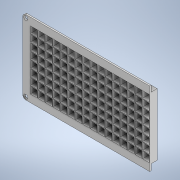
# Autodesk Inventor part: Grid
Saved by Autodesk Inventor 2020 (Build 240168000, 168)
## iProperties
Created: 2021-04-13
Part Number: Grid
Material: Generic
Document SubType Name: Modeling
Designer: user
Density: 1 g/cm^3
Appearance: Default
Author: user
Autodesk Inventor part; units mm, degrees
(part 1 of 2)
ref_plane "YZ Plane" through (0, 0, 0) normal (1, 0, 0) x (0, 1, 0)
ref_plane "XZ Plane" through (0, 0, 0) normal (0, 1, 0) x (-1, 0, 0)
ref_plane "XY Plane" through (0, 0, 0) normal (0, 0, 1) x (1, 0, 0)
sketch "Sketch4" plane through (0, 0, 0) normal (0, 0, 1) x (1, 0, 0)
  line L0 (0, 0) -> (5, 0)
  line L1 (5, 0) -> (5, 5)
  line L2 (5, 5) -> (0, 5)
  line L3 (0, 5) -> (0, 0)
  line L4 (-2, 7) -> (7, 7)
  line L5 (7, 7) -> (7, -2)
  line L6 (7, -2) -> (-2, -2)
  line L7 (-2, -2) -> (-2, 7)
  line L8 (10, 0) -> (15, 0)
  line L9 (15, 0) -> (15, 5)
  line L10 (15, 5) -> (10, 5)
  line L11 (10, 5) -> (10, 0)
  line L12 (20, 0) -> (25, 0)
  line L13 (25, 0) -> (25, 5)
  line L14 (25, 5) -> (20, 5)
  line L15 (20, 5) -> (20, 0)
  line L16 (30, 0) -> (35, 0)
  line L17 (35, 0) -> (35, 5)
  line L18 (35, 5) -> (30, 5)
  line L19 (30, 5) -> (30, 0)
  line L20 (40, 0) -> (45, 0)
  line L21 (45, 0) -> (45, 5)
  line L22 (45, 5) -> (40, 5)
  line L23 (40, 5) -> (40, 0)
  line L24 (50, 0) -> (55, 0)
  line L25 (55, 0) -> (55, 5)
  line L26 (55, 5) -> (50, 5)
  line L27 (50, 5) -> (50, 0)
  line L28 (60, 0) -> (65, 0)
  line L29 (65, 0) -> (65, 5)
  line L30 (65, 5) -> (60, 5)
  line L31 (60, 5) -> (60, 0)
  line L32 (70, 0) -> (75, 0)
  line L33 (75, 0) -> (75, 5)
  line L34 (75, 5) -> (70, 5)
  line L35 (70, 5) -> (70, 0)
  line L36 (80, 0) -> (85, 0)
  line L37 (85, 0) -> (85, 5)
  line L38 (85, 5) -> (80, 5)
  line L39 (80, 5) -> (80, 0)
  line L40 (90, 0) -> (95, 0)
  line L41 (95, 0) -> (95, 5)
  line L42 (95, 5) -> (90, 5)
  line L43 (90, 5) -> (90, 0)
  line L44 (100, 0) -> (105, 0)
  line L45 (105, 0) -> (105, 5)
  line L46 (105, 5) -> (100, 5)
  line L47 (100, 5) -> (100, 0)
  line L48 (110, 0) -> (115, 0)
  line L49 (115, 0) -> (115, 5)
  line L50 (115, 5) -> (110, 5)
  line L51 (110, 5) -> (110, 0)
  line L52 (120, 0) -> (125, 0)
  line L53 (125, 0) -> (125, 5)
  line L54 (125, 5) -> (120, 5)
  line L55 (120, 5) -> (120, 0)
  line L56 (130, 0) -> (135, 0)
  line L57 (135, 0) -> (135, 5)
  line L58 (135, 5) -> (130, 5)
  line L59 (130, 5) -> (130, 0)
  line L60 (140, 0) -> (145, 0)
  line L61 (145, 0) -> (145, 5)
  line L62 (145, 5) -> (140, 5)
  line L63 (140, 5) -> (140, 0)
  line L64 (150, 0) -> (155, 0)
  line L65 (155, 0) -> (155, 5)
  line L66 (155, 5) -> (150, 5)
  line L67 (150, 5) -> (150, 0)
  line L68 (160, 0) -> (165, 0)
  line L69 (165, 0) -> (165, 5)
  line L70 (165, 5) -> (160, 5)
  line L71 (160, 5) -> (160, 0)
  line L72 (170, 0) -> (175, 0)
  line L73 (175, 0) -> (175, 5)
  line L74 (175, 5) -> (170, 5)
  line L75 (170, 5) -> (170, 0)
  line L76 (180, 0) -> (185, 0)
  line L77 (185, 0) -> (185, 5)
  line L78 (185, 5) -> (180, 5)
  line L79 (180, 5) -> (180, 0)
  line L80 (190, 0) -> (195, 0)
  line L81 (195, 0) -> (195, 5)
  line L82 (195, 5) -> (190, 5)
  line L83 (190, 5) -> (190, 0)
  line L84 (200, 0) -> (205, 0)
  line L85 (205, 0) -> (205, 5)
  line L86 (205, 5) -> (200, 5)
  line L87 (200, 5) -> (200, 0)
  line L88 (210, 0) -> (215, 0)
  line L89 (215, 0) -> (215, 5)
  line L90 (215, 5) -> (210, 5)
  line L91 (210, 5) -> (210, 0)
  line L92 (220, 0) -> (225, 0)
  line L93 (225, 0) -> (225, 5)
  line L94 (225, 5) -> (220, 5)
  line L95 (220, 5) -> (220, 0)
  line L96 (230, 0) -> (235, 0)
  line L97 (235, 0) -> (235, 5)
  line L98 (235, 5) -> (230, 5)
  line L99 (230, 5) -> (230, 0)
  line L100 (240, 0) -> (245, 0)
  line L101 (245, 0) -> (245, 5)
  line L102 (245, 5) -> (240, 5)
  line L103 (240, 5) -> (240, 0)
  line L104 (250, 0) -> (255, 0)
  line L105 (255, 0) -> (255, 5)
  line L106 (255, 5) -> (250, 5)
  line L107 (250, 5) -> (250, 0)
  line L108 (260, 0) -> (265, 0)
  line L109 (265, 0) -> (265, 5)
  line L110 (265, 5) -> (260, 5)
  line L111 (260, 5) -> (260, 0)
  line L112 (270, 0) -> (275, 0)
  line L113 (275, 0) -> (275, 5)
  line L114 (275, 5) -> (270, 5)
  line L115 (270, 5) -> (270, 0)
  line L116 (280, 0) -> (285, 0)
  line L117 (285, 0) -> (285, 5)
  line L118 (285, 5) -> (280, 5)
  line L119 (280, 5) -> (280, 0)
  line L120 (290, 0) -> (295, 0)
  line L121 (295, 0) -> (295, 5)
  line L122 (295, 5) -> (290, 5)
  line L123 (290, 5) -> (290, 0)
  line L124 (300, 0) -> (305, 0)
  line L125 (305, 0) -> (305, 5)
  line L126 (305, 5) -> (300, 5)
  line L127 (300, 5) -> (300, 0)
  line L128 (310, 0) -> (315, 0)
  line L129 (315, 0) -> (315, 5)
  line L130 (315, 5) -> (310, 5)
  line L131 (310, 5) -> (310, 0)
  line L132 (0, -10) -> (5, -10)
  line L133 (5, -10) -> (5, -5)
  line L134 (5, -5) -> (0, -5)
  line L135 (0, -5) -> (0, -10)
  line L136 (10, -10) -> (15, -10)
  line L137 (15, -10) -> (15, -5)
  line L138 (15, -5) -> (10, -5)
  line L139 (10, -5) -> (10, -10)
  line L140 (20, -10) -> (25, -10)
  line L141 (25, -10) -> (25, -5)
  line L142 (25, -5) -> (20, -5)
  line L143 (20, -5) -> (20, -10)
  line L144 (30, -10) -> (35, -10)
  line L145 (35, -10) -> (35, -5)
  line L146 (35, -5) -> (30, -5)
  line L147 (30, -5) -> (30, -10)
  line L148 (40, -10) -> (45, -10)
  line L149 (45, -10) -> (45, -5)
  line L150 (45, -5) -> (40, -5)
  line L151 (40, -5) -> (40, -10)
  line L152 (50, -10) -> (55, -10)
  line L153 (55, -10) -> (55, -5)
  line L154 (55, -5) -> (50, -5)
  line L155 (50, -5) -> (50, -10)
  line L156 (60, -10) -> (65, -10)
  line L157 (65, -10) -> (65, -5)
  line L158 (65, -5) -> (60, -5)
  line L159 (60, -5) -> (60, -10)
  line L160 (70, -10) -> (75, -10)
  line L161 (75, -10) -> (75, -5)
  line L162 (75, -5) -> (70, -5)
  line L163 (70, -5) -> (70, -10)
  line L164 (80, -10) -> (85, -10)
  line L165 (85, -10) -> (85, -5)
  line L166 (85, -5) -> (80, -5)
  line L167 (80, -5) -> (80, -10)
  line L168 (90, -10) -> (95, -10)
  line L169 (95, -10) -> (95, -5)
  line L170 (95, -5) -> (90, -5)
  line L171 (90, -5) -> (90, -10)
  line L172 (100, -10) -> (105, -10)
  line L173 (105, -10) -> (105, -5)
  line L174 (105, -5) -> (100, -5)
  line L175 (100, -5) -> (100, -10)
  line L176 (110, -10) -> (115, -10)
  line L177 (115, -10) -> (115, -5)
  line L178 (115, -5) -> (110, -5)
  line L179 (110, -5) -> (110, -10)
  line L180 (120, -10) -> (125, -10)
  line L181 (125, -10) -> (125, -5)
  line L182 (125, -5) -> (120, -5)
  line L183 (120, -5) -> (120, -10)
  line L184 (130, -10) -> (135, -10)
  line L185 (135, -10) -> (135, -5)
  line L186 (135, -5) -> (130, -5)
  line L187 (130, -5) -> (130, -10)
  line L188 (140, -10) -> (145, -10)
  line L189 (145, -10) -> (145, -5)
  line L190 (145, -5) -> (140, -5)
  line L191 (140, -5) -> (140, -10)
  line L192 (150, -10) -> (155, -10)
  line L193 (155, -10) -> (155, -5)
  line L194 (155, -5) -> (150, -5)
  line L195 (150, -5) -> (150, -10)
  line L196 (160, -10) -> (165, -10)
  line L197 (165, -10) -> (165, -5)
  line L198 (165, -5) -> (160, -5)
  line L199 (160, -5) -> (160, -10)
  line L200 (170, -10) -> (175, -10)
  line L201 (175, -10) -> (175, -5)
  line L202 (175, -5) -> (170, -5)
  line L203 (170, -5) -> (170, -10)
  line L204 (180, -10) -> (185, -10)
  line L205 (185, -10) -> (185, -5)
  line L206 (185, -5) -> (180, -5)
  line L207 (180, -5) -> (180, -10)
  line L208 (190, -10) -> (195, -10)
  line L209 (195, -10) -> (195, -5)
  line L210 (195, -5) -> (190, -5)
  line L211 (190, -5) -> (190, -10)
  line L212 (200, -10) -> (205, -10)
  line L213 (205, -10) -> (205, -5)
  line L214 (205, -5) -> (200, -5)
  line L215 (200, -5) -> (200, -10)
  line L216 (210, -10) -> (215, -10)
  line L217 (215, -10) -> (215, -5)
  line L218 (215, -5) -> (210, -5)
  line L219 (210, -5) -> (210, -10)
  line L220 (220, -10) -> (225, -10)
  line L221 (225, -10) -> (225, -5)
  line L222 (225, -5) -> (220, -5)
  line L223 (220, -5) -> (220, -10)
  line L224 (230, -10) -> (235, -10)
  line L225 (235, -10) -> (235, -5)
  line L226 (235, -5) -> (230, -5)
  line L227 (230, -5) -> (230, -10)
  line L228 (240, -10) -> (245, -10)
  line L229 (245, -10) -> (245, -5)
  line L230 (245, -5) -> (240, -5)
  line L231 (240, -5) -> (240, -10)
  line L232 (250, -10) -> (255, -10)
  line L233 (255, -10) -> (255, -5)
  line L234 (255, -5) -> (250, -5)
  line L235 (250, -5) -> (250, -10)
  line L236 (260, -10) -> (265, -10)
  line L237 (265, -10) -> (265, -5)
  line L238 (265, -5) -> (260, -5)
  line L239 (260, -5) -> (260, -10)
  line L240 (270, -10) -> (275, -10)
  line L241 (275, -10) -> (275, -5)
  line L242 (275, -5) -> (270, -5)
  line L243 (270, -5) -> (270, -10)
  line L244 (280, -10) -> (285, -10)
  line L245 (285, -10) -> (285, -5)
  line L246 (285, -5) -> (280, -5)
  line L247 (280, -5) -> (280, -10)
  line L248 (290, -10) -> (295, -10)
  line L249 (295, -10) -> (295, -5)
  line L250 (295, -5) -> (290, -5)
  line L251 (290, -5) -> (290, -10)
  line L252 (300, -10) -> (305, -10)
  line L253 (305, -10) -> (305, -5)
  line L254 (305, -5) -> (300, -5)
  line L255 (300, -5) -> (300, -10)
  line L256 (310, -10) -> (315, -10)
  line L257 (315, -10) -> (315, -5)
  line L258 (315, -5) -> (310, -5)
  line L259 (310, -5) -> (310, -10)
  line L260 (0, -20) -> (5, -20)
  line L261 (5, -20) -> (5, -15)
  line L262 (5, -15) -> (0, -15)
  line L263 (0, -15) -> (0, -20)
  line L264 (10, -20) -> (15, -20)
  line L265 (15, -20) -> (15, -15)
  line L266 (15, -15) -> (10, -15)
  line L267 (10, -15) -> (10, -20)
  line L268 (20, -20) -> (25, -20)
  line L269 (25, -20) -> (25, -15)
  line L270 (25, -15) -> (20, -15)
  line L271 (20, -15) -> (20, -20)
  line L272 (30, -20) -> (35, -20)
  line L273 (35, -20) -> (35, -15)
  line L274 (35, -15) -> (30, -15)
  line L275 (30, -15) -> (30, -20)
  line L276 (40, -20) -> (45, -20)
  line L277 (45, -20) -> (45, -15)
  line L278 (45, -15) -> (40, -15)
  line L279 (40, -15) -> (40, -20)
  line L280 (50, -20) -> (55, -20)
  line L281 (55, -20) -> (55, -15)
  line L282 (55, -15) -> (50, -15)
  line L283 (50, -15) -> (50, -20)
  line L284 (60, -20) -> (65, -20)
  line L285 (65, -20) -> (65, -15)
  line L286 (65, -15) -> (60, -15)
  line L287 (60, -15) -> (60, -20)
  line L288 (70, -20) -> (75, -20)
  line L289 (75, -20) -> (75, -15)
  line L290 (75, -15) -> (70, -15)
  line L291 (70, -15) -> (70, -20)
  line L292 (80, -20) -> (85, -20)
  line L293 (85, -20) -> (85, -15)
  line L294 (85, -15) -> (80, -15)
  line L295 (80, -15) -> (80, -20)
  line L296 (90, -20) -> (95, -20)
  line L297 (95, -20) -> (95, -15)
  line L298 (95, -15) -> (90, -15)
  line L299 (90, -15) -> (90, -20)
  line L300 (100, -20) -> (105, -20)
  line L301 (105, -20) -> (105, -15)
  line L302 (105, -15) -> (100, -15)
  line L303 (100, -15) -> (100, -20)
  line L304 (110, -20) -> (115, -20)
  line L305 (115, -20) -> (115, -15)
  line L306 (115, -15) -> (110, -15)
  line L307 (110, -15) -> (110, -20)
  line L308 (120, -20) -> (125, -20)
  line L309 (125, -20) -> (125, -15)
  line L310 (125, -15) -> (120, -15)
  line L311 (120, -15) -> (120, -20)
  line L312 (130, -20) -> (135, -20)
  line L313 (135, -20) -> (135, -15)
  line L314 (135, -15) -> (130, -15)
  line L315 (130, -15) -> (130, -20)
  line L316 (140, -20) -> (145, -20)
  line L317 (145, -20) -> (145, -15)
  line L318 (145, -15) -> (140, -15)
  line L319 (140, -15) -> (140, -20)
  line L320 (150, -20) -> (155, -20)
  line L321 (155, -20) -> (155, -15)
  line L322 (155, -15) -> (150, -15)
  line L323 (150, -15) -> (150, -20)
  line L324 (160, -20) -> (165, -20)
  line L325 (165, -20) -> (165, -15)
  line L326 (165, -15) -> (160, -15)
  line L327 (160, -15) -> (160, -20)
  line L328 (170, -20) -> (175, -20)
  line L329 (175, -20) -> (175, -15)
  line L330 (175, -15) -> (170, -15)
  line L331 (170, -15) -> (170, -20)
  line L332 (180, -20) -> (185, -20)
  line L333 (185, -20) -> (185, -15)
  line L334 (185, -15) -> (180, -15)
  line L335 (180, -15) -> (180, -20)
  line L336 (190, -20) -> (195, -20)
  line L337 (195, -20) -> (195, -15)
  line L338 (195, -15) -> (190, -15)
  line L339 (190, -15) -> (190, -20)
  line L340 (200, -20) -> (205, -20)
  line L341 (205, -20) -> (205, -15)
  line L342 (205, -15) -> (200, -15)
  line L343 (200, -15) -> (200, -20)
  line L344 (210, -20) -> (215, -20)
  line L345 (215, -20) -> (215, -15)
  line L346 (215, -15) -> (210, -15)
  line L347 (210, -15) -> (210, -20)
  line L348 (220, -20) -> (225, -20)
  line L349 (225, -20) -> (225, -15)
  line L350 (225, -15) -> (220, -15)
  line L351 (220, -15) -> (220, -20)
  line L352 (230, -20) -> (235, -20)
  line L353 (235, -20) -> (235, -15)
  line L354 (235, -15) -> (230, -15)
  line L355 (230, -15) -> (230, -20)
  line L356 (240, -20) -> (245, -20)
  line L357 (245, -20) -> (245, -15)
  line L358 (245, -15) -> (240, -15)
  line L359 (240, -15) -> (240, -20)
  line L360 (250, -20) -> (255, -20)
  line L361 (255, -20) -> (255, -15)
  line L362 (255, -15) -> (250, -15)
  line L363 (250, -15) -> (250, -20)
  line L364 (260, -20) -> (265, -20)
  line L365 (265, -20) -> (265, -15)
  line L366 (265, -15) -> (260, -15)
  line L367 (260, -15) -> (260, -20)
  line L368 (270, -20) -> (275, -20)
  line L369 (275, -20) -> (275, -15)
  line L370 (275, -15) -> (270, -15)
  line L371 (270, -15) -> (270, -20)
  line L372 (280, -20) -> (285, -20)
  line L373 (285, -20) -> (285, -15)
  line L374 (285, -15) -> (280, -15)
  line L375 (280, -15) -> (280, -20)
  line L376 (290, -20) -> (295, -20)
  line L377 (295, -20) -> (295, -15)
  line L378 (295, -15) -> (290, -15)
  line L379 (290, -15) -> (290, -20)
  line L380 (300, -20) -> (305, -20)
  line L381 (305, -20) -> (305, -15)
  line L382 (305, -15) -> (300, -15)
  line L383 (300, -15) -> (300, -20)
  line L384 (310, -20) -> (315, -20)
  line L385 (315, -20) -> (315, -15)
  line L386 (315, -15) -> (310, -15)
  line L387 (310, -15) -> (310, -20)
  line L388 (0, -30) -> (5, -30)
  line L389 (5, -30) -> (5, -25)
  line L390 (5, -25) -> (0, -25)
  line L391 (0, -25) -> (0, -30)
  line L392 (10, -30) -> (15, -30)
  line L393 (15, -30) -> (15, -25)
  line L394 (15, -25) -> (10, -25)
  line L395 (10, -25) -> (10, -30)
  line L396 (20, -30) -> (25, -30)
  line L397 (25, -30) -> (25, -25)
  line L398 (25, -25) -> (20, -25)
  line L399 (20, -25) -> (20, -30)
  line L400 (30, -30) -> (35, -30)
  line L401 (35, -30) -> (35, -25)
  line L402 (35, -25) -> (30, -25)
  line L403 (30, -25) -> (30, -30)
  line L404 (40, -30) -> (45, -30)
  line L405 (45, -30) -> (45, -25)
  line L406 (45, -25) -> (40, -25)
  line L407 (40, -25) -> (40, -30)
  line L408 (50, -30) -> (55, -30)
  line L409 (55, -30) -> (55, -25)
  line L410 (55, -25) -> (50, -25)
  line L411 (50, -25) -> (50, -30)
  line L412 (60, -30) -> (65, -30)
  line L413 (65, -30) -> (65, -25)
  line L414 (65, -25) -> (60, -25)
  line L415 (60, -25) -> (60, -30)
  line L416 (70, -30) -> (75, -30)
  line L417 (75, -30) -> (75, -25)
  line L418 (75, -25) -> (70, -25)
  line L419 (70, -25) -> (70, -30)
  line L420 (80, -30) -> (85, -30)
  line L421 (85, -30) -> (85, -25)
  line L422 (85, -25) -> (80, -25)
  line L423 (80, -25) -> (80, -30)
  line L424 (90, -30) -> (95, -30)
  line L425 (95, -30) -> (95, -25)
  line L426 (95, -25) -> (90, -25)
  line L427 (90, -25) -> (90, -30)
  line L428 (100, -30) -> (105, -30)
  line L429 (105, -30) -> (105, -25)
  line L430 (105, -25) -> (100, -25)
  line L431 (100, -25) -> (100, -30)
  line L432 (110, -30) -> (115, -30)
  line L433 (115, -30) -> (115, -25)
  line L434 (115, -25) -> (110, -25)
  line L435 (110, -25) -> (110, -30)
  line L436 (120, -30) -> (125, -30)
  line L437 (125, -30) -> (125, -25)
  line L438 (125, -25) -> (120, -25)
  line L439 (120, -25) -> (120, -30)
  line L440 (130, -30) -> (135, -30)
  line L441 (135, -30) -> (135, -25)
  line L442 (135, -25) -> (130, -25)
  line L443 (130, -25) -> (130, -30)
  line L444 (140, -30) -> (145, -30)
  line L445 (145, -30) -> (145, -25)
  line L446 (145, -25) -> (140, -25)
  line L447 (140, -25) -> (140, -30)
  line L448 (150, -30) -> (155, -30)
  line L449 (155, -30) -> (155, -25)
  line L450 (155, -25) -> (150, -25)
  line L451 (150, -25) -> (150, -30)
  line L452 (160, -30) -> (165, -30)
  line L453 (165, -30) -> (165, -25)
  line L454 (165, -25) -> (160, -25)
  line L455 (160, -25) -> (160, -30)
  line L456 (170, -30) -> (175, -30)
  line L457 (175, -30) -> (175, -25)
  line L458 (175, -25) -> (170, -25)
  line L459 (170, -25) -> (170, -30)
  line L460 (180, -30) -> (185, -30)
  line L461 (185, -30) -> (185, -25)
  line L462 (185, -25) -> (180, -25)
  line L463 (180, -25) -> (180, -30)
  line L464 (190, -30) -> (195, -30)
  line L465 (195, -30) -> (195, -25)
  line L466 (195, -25) -> (190, -25)
  line L467 (190, -25) -> (190, -30)
  line L468 (200, -30) -> (205, -30)
  line L469 (205, -30) -> (205, -25)
  line L470 (205, -25) -> (200, -25)
  line L471 (200, -25) -> (200, -30)
  line L472 (210, -30) -> (215, -30)
  line L473 (215, -30) -> (215, -25)
  line L474 (215, -25) -> (210, -25)
  line L475 (210, -25) -> (210, -30)
  line L476 (220, -30) -> (225, -30)
  line L477 (225, -30) -> (225, -25)
  line L478 (225, -25) -> (220, -25)
  line L479 (220, -25) -> (220, -30)
  line L480 (230, -30) -> (235, -30)
  line L481 (235, -30) -> (235, -25)
  line L482 (235, -25) -> (230, -25)
  line L483 (230, -25) -> (230, -30)
  line L484 (240, -30) -> (245, -30)
  line L485 (245, -30) -> (245, -25)
  line L486 (245, -25) -> (240, -25)
  line L487 (240, -25) -> (240, -30)
  line L488 (250, -30) -> (255, -30)
  line L489 (255, -30) -> (255, -25)
  line L490 (255, -25) -> (250, -25)
  line L491 (250, -25) -> (250, -30)
  line L492 (260, -30) -> (265, -30)
  line L493 (265, -30) -> (265, -25)
  line L494 (265, -25) -> (260, -25)
  line L495 (260, -25) -> (260, -30)
  line L496 (270, -30) -> (275, -30)
  line L497 (275, -30) -> (275, -25)
  line L498 (275, -25) -> (270, -25)
  line L499 (270, -25) -> (270, -30)
  line L500 (280, -30) -> (285, -30)
  line L501 (285, -30) -> (285, -25)
  line L502 (285, -25) -> (280, -25)
  line L503 (280, -25) -> (280, -30)
  line L504 (290, -30) -> (295, -30)
  line L505 (295, -30) -> (295, -25)
  line L506 (295, -25) -> (290, -25)
  line L507 (290, -25) -> (290, -30)
  line L508 (300, -30) -> (305, -30)
  line L509 (305, -30) -> (305, -25)
  line L510 (305, -25) -> (300, -25)
  line L511 (300, -25) -> (300, -30)
  line L512 (310, -30) -> (315, -30)
  line L513 (315, -30) -> (315, -25)
  line L514 (315, -25) -> (310, -25)
  line L515 (310, -25) -> (310, -30)
  line L516 (0, -40) -> (5, -40)
  line L517 (5, -40) -> (5, -35)
  line L518 (5, -35) -> (0, -35)
  line L519 (0, -35) -> (0, -40)
  line L520 (10, -40) -> (15, -40)
  line L521 (15, -40) -> (15, -35)
  line L522 (15, -35) -> (10, -35)
  line L523 (10, -35) -> (10, -40)
  line L524 (20, -40) -> (25, -40)
  line L525 (25, -40) -> (25, -35)
  line L526 (25, -35) -> (20, -35)
  line L527 (20, -35) -> (20, -40)
  line L528 (30, -40) -> (35, -40)
  line L529 (35, -40) -> (35, -35)
  line L530 (35, -35) -> (30, -35)
  line L531 (30, -35) -> (30, -40)
  line L532 (40, -40) -> (45, -40)
  line L533 (45, -40) -> (45, -35)
  line L534 (45, -35) -> (40, -35)
  line L535 (40, -35) -> (40, -40)
  line L536 (50, -40) -> (55, -40)
  line L537 (55, -40) -> (55, -35)
  line L538 (55, -35) -> (50, -35)
  line L539 (50, -35) -> (50, -40)
  line L540 (60, -40) -> (65, -40)
  line L541 (65, -40) -> (65, -35)
  line L542 (65, -35) -> (60, -35)
  line L543 (60, -35) -> (60, -40)
  line L544 (70, -40) -> (75, -40)
  line L545 (75, -40) -> (75, -35)
  line L546 (75, -35) -> (70, -35)
  line L547 (70, -35) -> (70, -40)
  line L548 (80, -40) -> (85, -40)
  line L549 (85, -40) -> (85, -35)
  line L550 (85, -35) -> (80, -35)
  line L551 (80, -35) -> (80, -40)
  line L552 (90, -40) -> (95, -40)
  line L553 (95, -40) -> (95, -35)
  line L554 (95, -35) -> (90, -35)
  line L555 (90, -35) -> (90, -40)
  line L556 (100, -40) -> (105, -40)
  line L557 (105, -40) -> (105, -35)
  line L558 (105, -35) -> (100, -35)
  line L559 (100, -35) -> (100, -40)
  line L560 (110, -40) -> (115, -40)
  line L561 (115, -40) -> (115, -35)
  line L562 (115, -35) -> (110, -35)
  line L563 (110, -35) -> (110, -40)
  line L564 (120, -40) -> (125, -40)
  line L565 (125, -40) -> (125, -35)
  line L566 (125, -35) -> (120, -35)
  line L567 (120, -35) -> (120, -40)
  line L568 (130, -40) -> (135, -40)
  line L569 (135, -40) -> (135, -35)
  line L570 (135, -35) -> (130, -35)
  line L571 (130, -35) -> (130, -40)
  line L572 (140, -40) -> (145, -40)
  line L573 (145, -40) -> (145, -35)
  line L574 (145, -35) -> (140, -35)
  line L575 (140, -35) -> (140, -40)
  line L576 (150, -40) -> (155, -40)
  line L577 (155, -40) -> (155, -35)
  line L578 (155, -35) -> (150, -35)
  line L579 (150, -35) -> (150, -40)
  line L580 (160, -40) -> (165, -40)
  line L581 (165, -40) -> (165, -35)
  line L582 (165, -35) -> (160, -35)
  line L583 (160, -35) -> (160, -40)
  line L584 (170, -40) -> (175, -40)
  line L585 (175, -40) -> (175, -35)
  line L586 (175, -35) -> (170, -35)
  line L587 (170, -35) -> (170, -40)
  line L588 (180, -40) -> (185, -40)
  line L589 (185, -40) -> (185, -35)
  line L590 (185, -35) -> (180, -35)
  line L591 (180, -35) -> (180, -40)
  line L592 (190, -40) -> (195, -40)
  line L593 (195, -40) -> (195, -35)
  line L594 (195, -35) -> (190, -35)
  line L595 (190, -35) -> (190, -40)
  line L596 (200, -40) -> (205, -40)
  line L597 (205, -40) -> (205, -35)
  line L598 (205, -35) -> (200, -35)
  line L599 (200, -35) -> (200, -40)
  line L600 (210, -40) -> (215, -40)
  line L601 (215, -40) -> (215, -35)
  line L602 (215, -35) -> (210, -35)
  line L603 (210, -35) -> (210, -40)
  line L604 (220, -40) -> (225, -40)
  line L605 (225, -40) -> (225, -35)
  line L606 (225, -35) -> (220, -35)
  line L607 (220, -35) -> (220, -40)
  line L608 (230, -40) -> (235, -40)
  line L609 (235, -40) -> (235, -35)
  line L610 (235, -35) -> (230, -35)
  line L611 (230, -35) -> (230, -40)
  line L612 (240, -40) -> (245, -40)
  line L613 (245, -40) -> (245, -35)
  line L614 (245, -35) -> (240, -35)
  line L615 (240, -35) -> (240, -40)
  line L616 (250, -40) -> (255, -40)
  line L617 (255, -40) -> (255, -35)
  line L618 (255, -35) -> (250, -35)
  line L619 (250, -35) -> (250, -40)
  line L620 (260, -40) -> (265, -40)
  line L621 (265, -40) -> (265, -35)
  line L622 (265, -35) -> (260, -35)
  line L623 (260, -35) -> (260, -40)
  line L624 (270, -40) -> (275, -40)
  line L625 (275, -40) -> (275, -35)
  line L626 (275, -35) -> (270, -35)
  line L627 (270, -35) -> (270, -40)
  line L628 (280, -40) -> (285, -40)
  line L629 (285, -40) -> (285, -35)
  line L630 (285, -35) -> (280, -35)
  line L631 (280, -35) -> (280, -40)
  line L632 (290, -40) -> (295, -40)
  line L633 (295, -40) -> (295, -35)
  line L634 (295, -35) -> (290, -35)
  line L635 (290, -35) -> (290, -40)
  line L636 (300, -40) -> (305, -40)
  line L637 (305, -40) -> (305, -35)
  line L638 (305, -35) -> (300, -35)
  line L639 (300, -35) -> (300, -40)
  line L640 (310, -40) -> (315, -40)
  line L641 (315, -40) -> (315, -35)
  line L642 (315, -35) -> (310, -35)
  line L643 (310, -35) -> (310, -40)
  line L644 (0, -50) -> (5, -50)
  line L645 (5, -50) -> (5, -45)
  line L646 (5, -45) -> (0, -45)
  line L647 (0, -45) -> (0, -50)
  line L648 (10, -50) -> (15, -50)
  line L649 (15, -50) -> (15, -45)
  line L650 (15, -45) -> (10, -45)
  line L651 (10, -45) -> (10, -50)
  line L652 (20, -50) -> (25, -50)
  line L653 (25, -50) -> (25, -45)
  line L654 (25, -45) -> (20, -45)
  line L655 (20, -45) -> (20, -50)
  line L656 (30, -50) -> (35, -50)
  line L657 (35, -50) -> (35, -45)
  line L658 (35, -45) -> (30, -45)
  line L659 (30, -45) -> (30, -50)
  line L660 (40, -50) -> (45, -50)
  line L661 (45, -50) -> (45, -45)
  line L662 (45, -45) -> (40, -45)
  line L663 (40, -45) -> (40, -50)
  line L664 (50, -50) -> (55, -50)
  line L665 (55, -50) -> (55, -45)
  line L666 (55, -45) -> (50, -45)
  line L667 (50, -45) -> (50, -50)
  line L668 (60, -50) -> (65, -50)
  line L669 (65, -50) -> (65, -45)
  line L670 (65, -45) -> (60, -45)
  line L671 (60, -45) -> (60, -50)
  line L672 (70, -50) -> (75, -50)
  line L673 (75, -50) -> (75, -45)
  line L674 (75, -45) -> (70, -45)
  line L675 (70, -45) -> (70, -50)
  line L676 (80, -50) -> (85, -50)
  line L677 (85, -50) -> (85, -45)
  line L678 (85, -45) -> (80, -45)
  line L679 (80, -45) -> (80, -50)
  line L680 (90, -50) -> (95, -50)
  line L681 (95, -50) -> (95, -45)
  line L682 (95, -45) -> (90, -45)
  line L683 (90, -45) -> (90, -50)
  line L684 (100, -50) -> (105, -50)
  line L685 (105, -50) -> (105, -45)
  line L686 (105, -45) -> (100, -45)
  line L687 (100, -45) -> (100, -50)
  line L688 (110, -50) -> (115, -50)
  line L689 (115, -50) -> (115, -45)
  line L690 (115, -45) -> (110, -45)
  line L691 (110, -45) -> (110, -50)
  line L692 (120, -50) -> (125, -50)
  line L693 (125, -50) -> (125, -45)
  line L694 (125, -45) -> (120, -45)
  line L695 (120, -45) -> (120, -50)
  line L696 (130, -50) -> (135, -50)
  line L697 (135, -50) -> (135, -45)
  line L698 (135, -45) -> (130, -45)
  line L699 (130, -45) -> (130, -50)
  line L700 (140, -50) -> (145, -50)
  line L701 (145, -50) -> (145, -45)
  line L702 (145, -45) -> (140, -45)
  line L703 (140, -45) -> (140, -50)
  line L704 (150, -50) -> (155, -50)
  line L705 (155, -50) -> (155, -45)
  line L706 (155, -45) -> (150, -45)
  line L707 (150, -45) -> (150, -50)
  line L708 (160, -50) -> (165, -50)
  line L709 (165, -50) -> (165, -45)
  line L710 (165, -45) -> (160, -45)
  line L711 (160, -45) -> (160, -50)
  line L712 (170, -50) -> (175, -50)
  line L713 (175, -50) -> (175, -45)
  line L714 (175, -45) -> (170, -45)
  line L715 (170, -45) -> (170, -50)
  line L716 (180, -50) -> (185, -50)
  line L717 (185, -50) -> (185, -45)
  line L718 (185, -45) -> (180, -45)
  line L719 (180, -45) -> (180, -50)
  line L720 (190, -50) -> (195, -50)
  line L721 (195, -50) -> (195, -45)
  line L722 (195, -45) -> (190, -45)
  line L723 (190, -45) -> (190, -50)
  line L724 (200, -50) -> (205, -50)
  line L725 (205, -50) -> (205, -45)
  line L726 (205, -45) -> (200, -45)
  line L727 (200, -45) -> (200, -50)
  line L728 (210, -50) -> (215, -50)
  line L729 (215, -50) -> (215, -45)
  line L730 (215, -45) -> (210, -45)
  line L731 (210, -45) -> (210, -50)
  line L732 (220, -50) -> (225, -50)
  line L733 (225, -50) -> (225, -45)
  line L734 (225, -45) -> (220, -45)
  line L735 (220, -45) -> (220, -50)
  line L736 (230, -50) -> (235, -50)
  line L737 (235, -50) -> (235, -45)
  line L738 (235, -45) -> (230, -45)
  line L739 (230, -45) -> (230, -50)
  line L740 (240, -50) -> (245, -50)
  line L741 (245, -50) -> (245, -45)
  line L742 (245, -45) -> (240, -45)
  line L743 (240, -45) -> (240, -50)
  line L744 (250, -50) -> (255, -50)
  line L745 (255, -50) -> (255, -45)
  line L746 (255, -45) -> (250, -45)
  line L747 (250, -45) -> (250, -50)
  line L748 (260, -50) -> (265, -50)
  line L749 (265, -50) -> (265, -45)
  line L750 (265, -45) -> (260, -45)
  line L751 (260, -45) -> (260, -50)
  line L752 (270, -50) -> (275, -50)
  line L753 (275, -50) -> (275, -45)
  line L754 (275, -45) -> (270, -45)
  line L755 (270, -45) -> (270, -50)
  line L756 (280, -50) -> (285, -50)
  line L757 (285, -50) -> (285, -45)
  line L758 (285, -45) -> (280, -45)
  line L759 (280, -45) -> (280, -50)
  line L760 (290, -50) -> (295, -50)
  line L761 (295, -50) -> (295, -45)
  line L762 (295, -45) -> (290, -45)
  line L763 (290, -45) -> (290, -50)
  line L764 (300, -50) -> (305, -50)
  line L765 (305, -50) -> (305, -45)
  line L766 (305, -45) -> (300, -45)
  line L767 (300, -45) -> (300, -50)
  line L768 (310, -50) -> (315, -50)
  line L769 (315, -50) -> (315, -45)
  line L770 (315, -45) -> (310, -45)
  line L771 (310, -45) -> (310, -50)
  line L772 (0, -60) -> (5, -60)
  line L773 (5, -60) -> (5, -55)
  line L774 (5, -55) -> (0, -55)
  line L775 (0, -55) -> (0, -60)
  line L776 (10, -60) -> (15, -60)
  line L777 (15, -60) -> (15, -55)
  line L778 (15, -55) -> (10, -55)
  line L779 (10, -55) -> (10, -60)
  line L780 (20, -60) -> (25, -60)
  line L781 (25, -60) -> (25, -55)
  line L782 (25, -55) -> (20, -55)
  line L783 (20, -55) -> (20, -60)
  line L784 (30, -60) -> (35, -60)
  line L785 (35, -60) -> (35, -55)
  line L786 (35, -55) -> (30, -55)
  line L787 (30, -55) -> (30, -60)
  line L788 (40, -60) -> (45, -60)
  line L789 (45, -60) -> (45, -55)
  line L790 (45, -55) -> (40, -55)
  line L791 (40, -55) -> (40, -60)
  line L792 (50, -60) -> (55, -60)
  line L793 (55, -60) -> (55, -55)
  line L794 (55, -55) -> (50, -55)
  line L795 (50, -55) -> (50, -60)
  line L796 (60, -60) -> (65, -60)
  line L797 (65, -60) -> (65, -55)
  line L798 (65, -55) -> (60, -55)
  line L799 (60, -55) -> (60, -60)
  line L800 (70, -60) -> (75, -60)
  line L801 (75, -60) -> (75, -55)
  line L802 (75, -55) -> (70, -55)
  line L803 (70, -55) -> (70, -60)
  line L804 (80, -60) -> (85, -60)
  line L805 (85, -60) -> (85, -55)
  line L806 (85, -55) -> (80, -55)
  line L807 (80, -55) -> (80, -60)
  line L808 (90, -60) -> (95, -60)
  line L809 (95, -60) -> (95, -55)
  line L810 (95, -55) -> (90, -55)
  line L811 (90, -55) -> (90, -60)
  line L812 (100, -60) -> (105, -60)
  line L813 (105, -60) -> (105, -55)
  line L814 (105, -55) -> (100, -55)
  line L815 (100, -55) -> (100, -60)
  line L816 (110, -60) -> (115, -60)
  line L817 (115, -60) -> (115, -55)
  line L818 (115, -55) -> (110, -55)
  line L819 (110, -55) -> (110, -60)
  line L820 (120, -60) -> (125, -60)
  line L821 (125, -60) -> (125, -55)
  line L822 (125, -55) -> (120, -55)
  line L823 (120, -55) -> (120, -60)
  line L824 (130, -60) -> (135, -60)
  line L825 (135, -60) -> (135, -55)
  line L826 (135, -55) -> (130, -55)
  line L827 (130, -55) -> (130, -60)
  line L828 (140, -60) -> (145, -60)
  line L829 (145, -60) -> (145, -55)
  line L830 (145, -55) -> (140, -55)
  line L831 (140, -55) -> (140, -60)
  line L832 (150, -60) -> (155, -60)
  line L833 (155, -60) -> (155, -55)
  line L834 (155, -55) -> (150, -55)
  line L835 (150, -55) -> (150, -60)
  line L836 (160, -60) -> (165, -60)
  line L837 (165, -60) -> (165, -55)
  line L838 (165, -55) -> (160, -55)
  line L839 (160, -55) -> (160, -60)
  line L840 (170, -60) -> (175, -60)
  line L841 (175, -60) -> (175, -55)
  line L842 (175, -55) -> (170, -55)
  line L843 (170, -55) -> (170, -60)
  line L844 (180, -60) -> (185, -60)
  line L845 (185, -60) -> (185, -55)
  line L846 (185, -55) -> (180, -55)
  line L847 (180, -55) -> (180, -60)
  line L848 (190, -60) -> (195, -60)
  line L849 (195, -60) -> (195, -55)
  line L850 (195, -55) -> (190, -55)
  line L851 (190, -55) -> (190, -60)
  line L852 (200, -60) -> (205, -60)
  line L853 (205, -60) -> (205, -55)
  line L854 (205, -55) -> (200, -55)
  line L855 (200, -55) -> (200, -60)
  line L856 (210, -60) -> (215, -60)
  line L857 (215, -60) -> (215, -55)
  line L858 (215, -55) -> (210, -55)
  line L859 (210, -55) -> (210, -60)
  line L860 (220, -60) -> (225, -60)
  line L861 (225, -60) -> (225, -55)
  line L862 (225, -55) -> (220, -55)
  line L863 (220, -55) -> (220, -60)
  line L864 (230, -60) -> (235, -60)
  line L865 (235, -60) -> (235, -55)
  line L866 (235, -55) -> (230, -55)
  line L867 (230, -55) -> (230, -60)
  line L868 (240, -60) -> (245, -60)
  line L869 (245, -60) -> (245, -55)
  line L870 (245, -55) -> (240, -55)
  line L871 (240, -55) -> (240, -60)
  line L872 (250, -60) -> (255, -60)
  line L873 (255, -60) -> (255, -55)
  line L874 (255, -55) -> (250, -55)
  line L875 (250, -55) -> (250, -60)
  line L876 (260, -60) -> (265, -60)
  line L877 (265, -60) -> (265, -55)
  line L878 (265, -55) -> (260, -55)
  line L879 (260, -55) -> (260, -60)
  line L880 (270, -60) -> (275, -60)
  line L881 (275, -60) -> (275, -55)
  line L882 (275, -55) -> (270, -55)
  line L883 (270, -55) -> (270, -60)
  line L884 (280, -60) -> (285, -60)
  line L885 (285, -60) -> (285, -55)
  line L886 (285, -55) -> (280, -55)
  line L887 (280, -55) -> (280, -60)
  line L888 (290, -60) -> (295, -60)
  line L889 (295, -60) -> (295, -55)
  line L890 (295, -55) -> (290, -55)
  line L891 (290, -55) -> (290, -60)
  line L892 (300, -60) -> (305, -60)
  line L893 (305, -60) -> (305, -55)
  line L894 (305, -55) -> (300, -55)
  line L895 (300, -55) -> (300, -60)
  line L896 (310, -60) -> (315, -60)
  line L897 (315, -60) -> (315, -55)
  line L898 (315, -55) -> (310, -55)
  line L899 (310, -55) -> (310, -60)
  line L900 (0, -70) -> (5, -70)
  line L901 (5, -70) -> (5, -65)
  line L902 (5, -65) -> (0, -65)
  line L903 (0, -65) -> (0, -70)
  line L904 (10, -70) -> (15, -70)
  line L905 (15, -70) -> (15, -65)
  line L906 (15, -65) -> (10, -65)
  line L907 (10, -65) -> (10, -70)
  line L908 (20, -70) -> (25, -70)
  line L909 (25, -70) -> (25, -65)
  line L910 (25, -65) -> (20, -65)
  line L911 (20, -65) -> (20, -70)
  line L912 (30, -70) -> (35, -70)
  line L913 (35, -70) -> (35, -65)
  line L914 (35, -65) -> (30, -65)
  line L915 (30, -65) -> (30, -70)
  line L916 (40, -70) -> (45, -70)
  line L917 (45, -70) -> (45, -65)
  line L918 (45, -65) -> (40, -65)
  line L919 (40, -65) -> (40, -70)
  line L920 (50, -70) -> (55, -70)
  line L921 (55, -70) -> (55, -65)
  line L922 (55, -65) -> (50, -65)
  line L923 (50, -65) -> (50, -70)
  line L924 (60, -70) -> (65, -70)
  line L925 (65, -70) -> (65, -65)
  line L926 (65, -65) -> (60, -65)
  line L927 (60, -65) -> (60, -70)
  line L928 (70, -70) -> (75, -70)
  line L929 (75, -70) -> (75, -65)
  line L930 (75, -65) -> (70, -65)
  line L931 (70, -65) -> (70, -70)
  line L932 (80, -70) -> (85, -70)
  line L933 (85, -70) -> (85, -65)
  line L934 (85, -65) -> (80, -65)
  line L935 (80, -65) -> (80, -70)
  line L936 (90, -70) -> (95, -70)
  line L937 (95, -70) -> (95, -65)
  line L938 (95, -65) -> (90, -65)
  line L939 (90, -65) -> (90, -70)
  line L940 (100, -70) -> (105, -70)
  line L941 (105, -70) -> (105, -65)
  line L942 (105, -65) -> (100, -65)
  line L943 (100, -65) -> (100, -70)
  line L944 (110, -70) -> (115, -70)
  line L945 (115, -70) -> (115, -65)
  line L946 (115, -65) -> (110, -65)
  line L947 (110, -65) -> (110, -70)
  line L948 (120, -70) -> (125, -70)
  line L949 (125, -70) -> (125, -65)
  line L950 (125, -65) -> (120, -65)
  line L951 (120, -65) -> (120, -70)
  line L952 (130, -70) -> (135, -70)
  line L953 (135, -70) -> (135, -65)
  line L954 (135, -65) -> (130, -65)
  line L955 (130, -65) -> (130, -70)
  line L956 (140, -70) -> (145, -70)
  line L957 (145, -70) -> (145, -65)
  line L958 (145, -65) -> (140, -65)
  line L959 (140, -65) -> (140, -70)
  line L960 (150, -70) -> (155, -70)
  line L961 (155, -70) -> (155, -65)
  line L962 (155, -65) -> (150, -65)
  line L963 (150, -65) -> (150, -70)
  line L964 (160, -70) -> (165, -70)
  line L965 (165, -70) -> (165, -65)
  line L966 (165, -65) -> (160, -65)
  line L967 (160, -65) -> (160, -70)
  line L968 (170, -70) -> (175, -70)
  line L969 (175, -70) -> (175, -65)
  line L970 (175, -65) -> (170, -65)
  line L971 (170, -65) -> (170, -70)
  line L972 (180, -70) -> (185, -70)
  line L973 (185, -70) -> (185, -65)
  line L974 (185, -65) -> (180, -65)
  line L975 (180, -65) -> (180, -70)
  line L976 (190, -70) -> (195, -70)
  line L977 (195, -70) -> (195, -65)
  line L978 (195, -65) -> (190, -65)
  line L979 (190, -65) -> (190, -70)
  line L980 (200, -70) -> (205, -70)
  line L981 (205, -70) -> (205, -65)
  line L982 (205, -65) -> (200, -65)
  line L983 (200, -65) -> (200, -70)
  line L984 (210, -70) -> (215, -70)
  line L985 (215, -70) -> (215, -65)
  line L986 (215, -65) -> (210, -65)
  line L987 (210, -65) -> (210, -70)
  line L988 (220, -70) -> (225, -70)
  line L989 (225, -70) -> (225, -65)
  line L990 (225, -65) -> (220, -65)
  line L991 (220, -65) -> (220, -70)
  line L992 (230, -70) -> (235, -70)
  line L993 (235, -70) -> (235, -65)
  line L994 (235, -65) -> (230, -65)
  line L995 (230, -65) -> (230, -70)
  line L996 (240, -70) -> (245, -70)
  line L997 (245, -70) -> (245, -65)
  line L998 (245, -65) -> (240, -65)
  line L999 (240, -65) -> (240, -70)
  line L1000 (250, -70) -> (255, -70)
  line L1001 (255, -70) -> (255, -65)
  line L1002 (255, -65) -> (250, -65)
  line L1003 (250, -65) -> (250, -70)
  line L1004 (260, -70) -> (265, -70)
  line L1005 (265, -70) -> (265, -65)
  line L1006 (265, -65) -> (260, -65)
  line L1007 (260, -65) -> (260, -70)
  line L1008 (270, -70) -> (275, -70)
  line L1009 (275, -70) -> (275, -65)
  line L1010 (275, -65) -> (270, -65)
  line L1011 (270, -65) -> (270, -70)
  line L1012 (280, -70) -> (285, -70)
  line L1013 (285, -70) -> (285, -65)
  line L1014 (285, -65) -> (280, -65)
  line L1015 (280, -65) -> (280, -70)
  line L1016 (290, -70) -> (295, -70)
  line L1017 (295, -70) -> (295, -65)
  line L1018 (295, -65) -> (290, -65)
  line L1019 (290, -65) -> (290, -70)
  line L1020 (300, -70) -> (305, -70)
  line L1021 (305, -70) -> (305, -65)
  line L1022 (305, -65) -> (300, -65)
  line L1023 (300, -65) -> (300, -70)
  line L1024 (310, -70) -> (315, -70)
  line L1025 (315, -70) -> (315, -65)
  line L1026 (315, -65) -> (310, -65)
  line L1027 (310, -65) -> (310, -70)
  line L1028 (8, 7) -> (17, 7)
  line L1029 (8, -2) -> (8, 7)
  line L1030 (17, -2) -> (8, -2)
  line L1031 (17, 7) -> (17, -2)
  line L1032 (18, 7) -> (27, 7)
  line L1033 (18, -2) -> (18, 7)
  line L1034 (27, -2) -> (18, -2)
  line L1035 (27, 7) -> (27, -2)
  line L1036 (28, 7) -> (37, 7)
  line L1037 (28, -2) -> (28, 7)
  line L1038 (37, -2) -> (28, -2)
  line L1039 (37, 7) -> (37, -2)
  line L1040 (38, 7) -> (47, 7)
  line L1041 (38, -2) -> (38, 7)
  line L1042 (47, -2) -> (38, -2)
  line L1043 (47, 7) -> (47, -2)
  line L1044 (48, 7) -> (57, 7)
  line L1045 (48, -2) -> (48, 7)
  line L1046 (57, -2) -> (48, -2)
  line L1047 (57, 7) -> (57, -2)
  line L1048 (58, 7) -> (67, 7)
  line L1049 (58, -2) -> (58, 7)
  line L1050 (67, -2) -> (58, -2)
  line L1051 (67, 7) -> (67, -2)
  line L1052 (68, 7) -> (77, 7)
  line L1053 (68, -2) -> (68, 7)
  line L1054 (77, -2) -> (68, -2)
  line L1055 (77, 7) -> (77, -2)
  line L1056 (78, 7) -> (87, 7)
  line L1057 (78, -2) -> (78, 7)
  line L1058 (87, -2) -> (78, -2)
  line L1059 (87, 7) -> (87, -2)
  line L1060 (88, 7) -> (97, 7)
  line L1061 (88, -2) -> (88, 7)
  line L1062 (97, -2) -> (88, -2)
  line L1063 (97, 7) -> (97, -2)
  line L1064 (98, 7) -> (107, 7)
  line L1065 (98, -2) -> (98, 7)
  line L1066 (107, -2) -> (98, -2)
  line L1067 (107, 7) -> (107, -2)
  line L1068 (108, 7) -> (117, 7)
  line L1069 (108, -2) -> (108, 7)
  line L1070 (117, -2) -> (108, -2)
  line L1071 (117, 7) -> (117, -2)
  line L1072 (118, 7) -> (127, 7)
  line L1073 (118, -2) -> (118, 7)
  line L1074 (127, -2) -> (118, -2)
  line L1075 (127, 7) -> (127, -2)
  line L1076 (128, 7) -> (137, 7)
  line L1077 (128, -2) -> (128, 7)
  line L1078 (137, -2) -> (128, -2)
  line L1079 (137, 7) -> (137, -2)
  line L1080 (138, 7) -> (147, 7)
  line L1081 (138, -2) -> (138, 7)
  line L1082 (147, -2) -> (138, -2)
  line L1083 (147, 7) -> (147, -2)
  line L1084 (148, 7) -> (157, 7)
  line L1085 (148, -2) -> (148, 7)
  line L1086 (157, -2) -> (148, -2)
  line L1087 (157, 7) -> (157, -2)
  line L1088 (158, 7) -> (167, 7)
  line L1089 (158, -2) -> (158, 7)
  line L1090 (167, -2) -> (158, -2)
  line L1091 (167, 7) -> (167, -2)
  line L1092 (168, 7) -> (177, 7)
  line L1093 (168, -2) -> (168, 7)
  line L1094 (177, -2) -> (168, -2)
  line L1095 (177, 7) -> (177, -2)
  line L1096 (178, 7) -> (187, 7)
  line L1097 (178, -2) -> (178, 7)
  line L1098 (187, -2) -> (178, -2)
  line L1099 (187, 7) -> (187, -2)
  line L1100 (188, 7) -> (197, 7)
  line L1101 (188, -2) -> (188, 7)
  line L1102 (197, -2) -> (188, -2)
  line L1103 (197, 7) -> (197, -2)
  line L1104 (198, 7) -> (207, 7)
  line L1105 (198, -2) -> (198, 7)
  line L1106 (207, -2) -> (198, -2)
  line L1107 (207, 7) -> (207, -2)
  line L1108 (208, 7) -> (217, 7)
  line L1109 (208, -2) -> (208, 7)
  line L1110 (217, -2) -> (208, -2)
  line L1111 (217, 7) -> (217, -2)
  line L1112 (218, 7) -> (227, 7)
  line L1113 (218, -2) -> (218, 7)
  line L1114 (227, -2) -> (218, -2)
  line L1115 (227, 7) -> (227, -2)
  line L1116 (228, 7) -> (237, 7)
  line L1117 (228, -2) -> (228, 7)
  line L1118 (237, -2) -> (228, -2)
  line L1119 (237, 7) -> (237, -2)
  line L1120 (238, 7) -> (247, 7)
  line L1121 (238, -2) -> (238, 7)
  line L1122 (247, -2) -> (238, -2)
  line L1123 (247, 7) -> (247, -2)
  line L1124 (248, 7) -> (257, 7)
  line L1125 (248, -2) -> (248, 7)
  line L1126 (257, -2) -> (248, -2)
  line L1127 (257, 7) -> (257, -2)
  line L1128 (258, 7) -> (267, 7)
  line L1129 (258, -2) -> (258, 7)
  line L1130 (267, -2) -> (258, -2)
  line L1131 (267, 7) -> (267, -2)
  line L1132 (268, 7) -> (277, 7)
  line L1133 (268, -2) -> (268, 7)
  line L1134 (277, -2) -> (268, -2)
  line L1135 (277, 7) -> (277, -2)
  line L1136 (278, 7) -> (287, 7)
  line L1137 (278, -2) -> (278, 7)
  line L1138 (287, -2) -> (278, -2)
  line L1139 (287, 7) -> (287, -2)
  line L1140 (288, 7) -> (297, 7)
  line L1141 (288, -2) -> (288, 7)
  line L1142 (297, -2) -> (288, -2)
  line L1143 (297, 7) -> (297, -2)
  line L1144 (298, 7) -> (307, 7)
  line L1145 (298, -2) -> (298, 7)
  line L1146 (307, -2) -> (298, -2)
  line L1147 (307, 7) -> (307, -2)
  line L1148 (308, 7) -> (317, 7)
  line L1149 (308, -2) -> (308, 7)
  line L1150 (317, -2) -> (308, -2)
  line L1151 (317, 7) -> (317, -2)
  line L1152 (-2, -3) -> (7, -3)
  line L1153 (-2, -12) -> (-2, -3)
  line L1154 (7, -12) -> (-2, -12)
  line L1155 (7, -3) -> (7, -12)
  line L1156 (8, -3) -> (17, -3)
  line L1157 (8, -12) -> (8, -3)
  line L1158 (17, -12) -> (8, -12)
  line L1159 (17, -3) -> (17, -12)
  line L1160 (18, -3) -> (27, -3)
  line L1161 (18, -12) -> (18, -3)
  line L1162 (27, -12) -> (18, -12)
  line L1163 (27, -3) -> (27, -12)
  line L1164 (28, -3) -> (37, -3)
  line L1165 (28, -12) -> (28, -3)
  line L1166 (37, -12) -> (28, -12)
  line L1167 (37, -3) -> (37, -12)
  line L1168 (38, -3) -> (47, -3)
  line L1169 (38, -12) -> (38, -3)
  line L1170 (47, -12) -> (38, -12)
  line L1171 (47, -3) -> (47, -12)
  line L1172 (48, -3) -> (57, -3)
  line L1173 (48, -12) -> (48, -3)
  line L1174 (57, -12) -> (48, -12)
  line L1175 (57, -3) -> (57, -12)
  line L1176 (58, -3) -> (67, -3)
  line L1177 (58, -12) -> (58, -3)
  line L1178 (67, -12) -> (58, -12)
  line L1179 (67, -3) -> (67, -12)
  line L1180 (68, -3) -> (77, -3)
  line L1181 (68, -12) -> (68, -3)
  line L1182 (77, -12) -> (68, -12)
  line L1183 (77, -3) -> (77, -12)
  line L1184 (78, -3) -> (87, -3)
  line L1185 (78, -12) -> (78, -3)
  line L1186 (87, -12) -> (78, -12)
  line L1187 (87, -3) -> (87, -12)
  line L1188 (88, -3) -> (97, -3)
  line L1189 (88, -12) -> (88, -3)
  line L1190 (97, -12) -> (88, -12)
  line L1191 (97, -3) -> (97, -12)
  line L1192 (98, -3) -> (107, -3)
  line L1193 (98, -12) -> (98, -3)
  line L1194 (107, -12) -> (98, -12)
  line L1195 (107, -3) -> (107, -12)
  line L1196 (108, -3) -> (117, -3)
  line L1197 (108, -12) -> (108, -3)
  line L1198 (117, -12) -> (108, -12)
  line L1199 (117, -3) -> (117, -12)
  line L1200 (118, -3) -> (127, -3)
  line L1201 (118, -12) -> (118, -3)
  line L1202 (127, -12) -> (118, -12)
  line L1203 (127, -3) -> (127, -12)
  line L1204 (128, -3) -> (137, -3)
  line L1205 (128, -12) -> (128, -3)
  line L1206 (137, -12) -> (128, -12)
  line L1207 (137, -3) -> (137, -12)
  line L1208 (138, -3) -> (147, -3)
  line L1209 (138, -12) -> (138, -3)
  line L1210 (147, -12) -> (138, -12)
  line L1211 (147, -3) -> (147, -12)
  line L1212 (148, -3) -> (157, -3)
  line L1213 (148, -12) -> (148, -3)
  line L1214 (157, -12) -> (148, -12)
  line L1215 (157, -3) -> (157, -12)
  line L1216 (158, -3) -> (167, -3)
  line L1217 (158, -12) -> (158, -3)
  line L1218 (167, -12) -> (158, -12)
  line L1219 (167, -3) -> (167, -12)
  line L1220 (168, -3) -> (177, -3)
  line L1221 (168, -12) -> (168, -3)
  line L1222 (177, -12) -> (168, -12)
  line L1223 (177, -3) -> (177, -12)
  line L1224 (178, -3) -> (187, -3)
  line L1225 (178, -12) -> (178, -3)
  line L1226 (187, -12) -> (178, -12)
  line L1227 (187, -3) -> (187, -12)
  line L1228 (188, -3) -> (197, -3)
  line L1229 (188, -12) -> (188, -3)
  line L1230 (197, -12) -> (188, -12)
  line L1231 (197, -3) -> (197, -12)
  line L1232 (198, -3) -> (207, -3)
  line L1233 (198, -12) -> (198, -3)
  line L1234 (207, -12) -> (198, -12)
  line L1235 (207, -3) -> (207, -12)
  line L1236 (208, -3) -> (217, -3)
  line L1237 (208, -12) -> (208, -3)
  line L1238 (217, -12) -> (208, -12)
  line L1239 (217, -3) -> (217, -12)
  line L1240 (218, -3) -> (227, -3)
  line L1241 (218, -12) -> (218, -3)
  line L1242 (227, -12) -> (218, -12)
  line L1243 (227, -3) -> (227, -12)
  line L1244 (228, -3) -> (237, -3)
  line L1245 (228, -12) -> (228, -3)
  line L1246 (237, -12) -> (228, -12)
  line L1247 (237, -3) -> (237, -12)
  line L1248 (238, -3) -> (247, -3)
  line L1249 (238, -12) -> (238, -3)
  line L1250 (247, -12) -> (238, -12)
  line L1251 (247, -3) -> (247, -12)
  line L1252 (248, -3) -> (257, -3)
  line L1253 (248, -12) -> (248, -3)
  line L1254 (257, -12) -> (248, -12)
  line L1255 (257, -3) -> (257, -12)
  line L1256 (258, -3) -> (267, -3)
  line L1257 (258, -12) -> (258, -3)
  line L1258 (267, -12) -> (258, -12)
  line L1259 (267, -3) -> (267, -12)
  line L1260 (268, -3) -> (277, -3)
  line L1261 (268, -12) -> (268, -3)
  line L1262 (277, -12) -> (268, -12)
  line L1263 (277, -3) -> (277, -12)
  line L1264 (278, -3) -> (287, -3)
  line L1265 (278, -12) -> (278, -3)
  line L1266 (287, -12) -> (278, -12)
  line L1267 (287, -3) -> (287, -12)
  line L1268 (288, -3) -> (297, -3)
  line L1269 (288, -12) -> (288, -3)
  line L1270 (297, -12) -> (288, -12)
  line L1271 (297, -3) -> (297, -12)
  line L1272 (298, -3) -> (307, -3)
  line L1273 (298, -12) -> (298, -3)
  line L1274 (307, -12) -> (298, -12)
  line L1275 (307, -3) -> (307, -12)
  line L1276 (308, -3) -> (317, -3)
  line L1277 (308, -12) -> (308, -3)
  line L1278 (317, -12) -> (308, -12)
  line L1279 (317, -3) -> (317, -12)
  line L1280 (-2, -13) -> (7, -13)
  line L1281 (-2, -22) -> (-2, -13)
  line L1282 (7, -22) -> (-2, -22)
  line L1283 (7, -13) -> (7, -22)
  line L1284 (8, -13) -> (17, -13)
  line L1285 (8, -22) -> (8, -13)
  line L1286 (17, -22) -> (8, -22)
  line L1287 (17, -13) -> (17, -22)
  line L1288 (18, -13) -> (27, -13)
  line L1289 (18, -22) -> (18, -13)
  line L1290 (27, -22) -> (18, -22)
  line L1291 (27, -13) -> (27, -22)
  line L1292 (28, -13) -> (37, -13)
  line L1293 (28, -22) -> (28, -13)
  line L1294 (37, -22) -> (28, -22)
  line L1295 (37, -13) -> (37, -22)
  line L1296 (38, -13) -> (47, -13)
  line L1297 (38, -22) -> (38, -13)
  line L1298 (47, -22) -> (38, -22)
  line L1299 (47, -13) -> (47, -22)
  line L1300 (48, -13) -> (57, -13)
  line L1301 (48, -22) -> (48, -13)
  line L1302 (57, -22) -> (48, -22)
  line L1303 (57, -13) -> (57, -22)
  line L1304 (58, -13) -> (67, -13)
  line L1305 (58, -22) -> (58, -13)
  line L1306 (67, -22) -> (58, -22)
  line L1307 (67, -13) -> (67, -22)
  line L1308 (68, -13) -> (77, -13)
  line L1309 (68, -22) -> (68, -13)
  line L1310 (77, -22) -> (68, -22)
  line L1311 (77, -13) -> (77, -22)
  line L1312 (78, -13) -> (87, -13)
  line L1313 (78, -22) -> (78, -13)
  line L1314 (87, -22) -> (78, -22)
  line L1315 (87, -13) -> (87, -22)
  line L1316 (88, -13) -> (97, -13)
  line L1317 (88, -22) -> (88, -13)
  line L1318 (97, -22) -> (88, -22)
  line L1319 (97, -13) -> (97, -22)
  line L1320 (98, -13) -> (107, -13)
  line L1321 (98, -22) -> (98, -13)
  line L1322 (107, -22) -> (98, -22)
  line L1323 (107, -13) -> (107, -22)
  line L1324 (108, -13) -> (117, -13)
  line L1325 (108, -22) -> (108, -13)
  line L1326 (117, -22) -> (108, -22)
  line L1327 (117, -13) -> (117, -22)
  line L1328 (118, -13) -> (127, -13)
  line L1329 (118, -22) -> (118, -13)
  line L1330 (127, -22) -> (118, -22)
  line L1331 (127, -13) -> (127, -22)
  line L1332 (128, -13) -> (137, -13)
  line L1333 (128, -22) -> (128, -13)
  line L1334 (137, -22) -> (128, -22)
  line L1335 (137, -13) -> (137, -22)
  line L1336 (138, -13) -> (147, -13)
  line L1337 (138, -22) -> (138, -13)
  line L1338 (147, -22) -> (138, -22)
  line L1339 (147, -13) -> (147, -22)
  line L1340 (148, -13) -> (157, -13)
  line L1341 (148, -22) -> (148, -13)
  line L1342 (157, -22) -> (148, -22)
  line L1343 (157, -13) -> (157, -22)
  line L1344 (158, -13) -> (167, -13)
  line L1345 (158, -22) -> (158, -13)
  line L1346 (167, -22) -> (158, -22)
  line L1347 (167, -13) -> (167, -22)
  line L1348 (168, -13) -> (177, -13)
  line L1349 (168, -22) -> (168, -13)
  line L1350 (177, -22) -> (168, -22)
  line L1351 (177, -13) -> (177, -22)
  line L1352 (178, -13) -> (187, -13)
  line L1353 (178, -22) -> (178, -13)
  line L1354 (187, -22) -> (178, -22)
  line L1355 (187, -13) -> (187, -22)
  line L1356 (188, -13) -> (197, -13)
  line L1357 (188, -22) -> (188, -13)
  line L1358 (197, -22) -> (188, -22)
  line L1359 (197, -13) -> (197, -22)
  line L1360 (198, -13) -> (207, -13)
  line L1361 (198, -22) -> (198, -13)
  line L1362 (207, -22) -> (198, -22)
  line L1363 (207, -13) -> (207, -22)
  line L1364 (208, -13) -> (217, -13)
  line L1365 (208, -22) -> (208, -13)
  line L1366 (217, -22) -> (208, -22)
  line L1367 (217, -13) -> (217, -22)
  line L1368 (218, -13) -> (227, -13)
  line L1369 (218, -22) -> (218, -13)
  line L1370 (227, -22) -> (218, -22)
  line L1371 (227, -13) -> (227, -22)
  line L1372 (228, -13) -> (237, -13)
  line L1373 (228, -22) -> (228, -13)
  line L1374 (237, -22) -> (228, -22)
  line L1375 (237, -13) -> (237, -22)
  line L1376 (238, -13) -> (247, -13)
  line L1377 (238, -22) -> (238, -13)
  line L1378 (247, -22) -> (238, -22)
  line L1379 (247, -13) -> (247, -22)
  line L1380 (248, -13) -> (257, -13)
  line L1381 (248, -22) -> (248, -13)
  line L1382 (257, -22) -> (248, -22)
  line L1383 (257, -13) -> (257, -22)